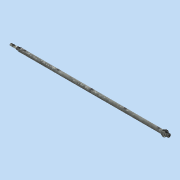
# Autodesk Inventor part: Spindel
Saved by Autodesk Inventor 2021 (Build 250183000, 183)
## iProperties
Created: 2024-03-13
Part Number: Spindel
Material: Generic
Document SubType Name: Modeling
Designer: Nokia
Density: 1 g/cm^3
Appearance: Formwork Holes
Author: Nokia
Autodesk Inventor part; units mm, degrees
ref_plane "YZ Plane" through (0, 0, 0) normal (1, 0, 0) x (0, 1, 0)
ref_plane "XZ Plane" through (0, 0, 0) normal (0, 1, 0) x (-1, 0, 0)
ref_plane "XY Plane" through (0, 0, 0) normal (0, 0, 1) x (1, 0, 0)
sketch "Sketch1" plane through (0, 0, 0) normal (0, 0, 1) x (1, 0, 0)
  line L0 (-1227.0505, 16) -> (-1227.0505, 12.5)
  arc A0 (72.9495, 16) -> (73.9495, 16) centre (73.4495, 16) ccw
  line L1 (73.9495, 16) -> (73.9495, 20)
  line L2 (73.9495, 20) -> (85.9495, 20)
  arc A1 (85.9495, 20) -> (86.9495, 20) centre (86.4495, 20) ccw
  line L3 (86.9495, 20) -> (86.9495, 26)
  line L4 (86.9495, 26) -> (98.9495, 26)
  line L5 (98.9495, 26) -> (98.9495, 15)
  arc A2 (98.9495, 15) -> (99.9495, 15) centre (99.4495, 15) ccw
  line L6 (99.9495, 15) -> (113.9495, 15)
  line L7 (-1310.4505, 0) -> (129.9495, 0)
  line L8 (-1598.5305, 0) -> (418.0295, 0) projected
  arc A3 (113.9495, 15) -> (114.9495, 15) centre (114.4495, 15) ccw
  line L9 (114.9495, 15) -> (129.9495, 15)
  line L10 (129.9495, 15) -> (129.9495, 0)
  arc A4 (-1228.0505, 12.5) -> (-1227.0505, 12.5) centre (-1227.5505, 12.5) ccw
  line L11 (-1228.0505, 12.5) -> (-1238.0505, 12.5)
  arc A5 (-1239.0505, 12.5) -> (-1238.0505, 12.5) centre (-1238.5505, 12.5) ccw
  line L12 (-1239.0505, 12.5) -> (-1251.0505, 12.5)
  line L13 (-1251.0505, 12.5) -> (-1251.0505, 10)
  line L14 (-1251.0505, 10) -> (-1310.4505, 10)
  line L15 (-1310.4505, 10) -> (-1310.4505, 0)
  arc A6 (-1219.0505, 16) -> (-1218.0505, 16) centre (-1218.5505, 16) ccw
  line L16 (72.9495, 16) -> (-1218.0505, 16)
  line L17 (-1227.0505, 16) -> (-1219.0505, 16)
  point P0 (0, 0)
  dimension "d6" = 12
  dimension "d9" = 12
  dimension "d29" = 0.5
  dimension "d30" = 0.5
  dimension "d32" = 15
  dimension "d44" = 20
  dimension "d46" = 26
  dimension "d52" = 15
  dimension "d57" = 0.5
  dimension "d58" = 10
  dimension "d62" = 2.5
  dimension "d63" = 59.4
  dimension "d70" = 1300
  dimension "d104" = 10
  dimension "d105" = 12.5
  dimension "d106" = 12.5
  dimension "d111" = 1291
  dimension "d112" = 0.5
  dimension "d113" = 0.5
  dimension "d114" = 4
  dimension "d121" = 0.5
  dimension "d122" = 0.5
  dimension "d123" = 31
  constraints: 34 end point, 14 point on circle, 7 centre point, 7 horizontal, 5 perpendicular, 4 point on line, 3 vertical
  measures "d6" distance of L1.end L2.end
  measures "d9" distance of L3.end L4.end
  measures "d29" radius of A2
  measures "d30" radius of A1
  measures "d32" distance of L9.start L9.end
  measures "d44" distance between parallel lines of L7 L2
  measures "d46" distance between parallel lines of L7 L4
  measures "d52" distance between parallel lines of L8 L9
  measures "d57" radius of A4
  measures "d58" distance of L11.start L11.end
  measures "d62" distance of L12.end L13.end
  measures "d63" distance of L13.end L14.end
  measures "d70" distance of L16.start L0.start
  measures "d104" distance of L14.end L7.start
  measures "d105" distance between parallel lines of L8 L11
  measures "d106" distance from line of L8 A4.centre
  measures "d111" distance of L16.start L16.end
  measures "d112" radius of A6
  measures "d113" radius of A0
  measures "d114" distance of L1.start L1.end
  measures "d121" radius of A5
  measures "d122" radius of A3
  measures "d123" distance between parallel lines of L5 L10
revolve "Revolution2" add sketch "Sketch1" angle 360 about axis through (-10, 0, 0) along (1, 0, 0)
chamfer "Chamfer1" distance 2 angle 45 2 edges at (98.9495, -26, 0) (86.9495, -26, 0)
thread "Thread2" size "M36x4" class "6g" standard "ANSI Metric M Profile" full length
chamfer "Chamfer2" distance 2 angle 45 1 edges at (129.9495, -15, 0)
sketch "Sketch4" plane through (129.9495, 0, 0) normal (1, 0, 0) x (0, 0, -1)
  circle A0 centre (0, 0) radius 15 projected
  line L0 (-2.5, 15) -> (2.5, 15)
  line L1 (2.5, 15) -> (2.5, 11)
  line L2 (2.5, 11) -> (-2.5, 11)
  line L3 (-2.5, 11) -> (-2.5, 15)
  point P0 (2.5, 14.7902)
  point P1 (-2.5, 14.7902)
  dimension "d47" = 4
  dimension "d49" = 5
  constraints: 8 end point, 2 horizontal, 2 perpendicular, 1 tangent
  measures "d47" distance of L0.end L1.end
  measures "d49" distance of L1.end L2.end
extrude "Extrusion3" cut sketch "Sketch4" against normal blind 16 contours L1 L2 L3 A0 picked at (0, 12.3333)
thread "Thread4" size "M30x3.5" class "6g" standard "ANSI Metric M Profile" full length
thread "Thread5" size "M25x2" class "6g" standard "ANSI Metric M Profile" full length
sketch "Sketch5" plane through (-1251.0505, 0, 0) normal (-1, 0, 0) x (0, 0, 1)
  circle A0 centre (0, 0) radius 12.5 projected
  line L0 (-2.5, 12.5) -> (2.5, 12.5)
  line L1 (2.5, 12.5) -> (2.5, 9.5)
  line L2 (2.5, 9.5) -> (-2.5, 9.5)
  line L3 (-2.5, 9.5) -> (-2.5, 12.5)
  line L4 (-2.5, 12.7574) -> (-2.5, 11) projected
  point P0 (2.5, 12.2474)
  point P1 (-2.5, 12.2474)
  dimension "d66" = 3
  dimension "d67" = 5
  constraints: 8 end point, 1 horizontal, 1 perpendicular, 1 point on line, 1 tangent
  measures "d66" distance of L0.end L1.end
  measures "d67" distance of L1.end L2.end
extrude "Extrusion4" cut sketch "Sketch5" against normal blind 13 contours L1 L2 L3 A0 picked at (0, 10.5)
chamfer "Chamfer4" distance 1 angle 45 1 edges at (73.9495, -20, 0)
chamfer "Chamfer5" distance 2 angle 45 1 edges at (-1310.4505, -10, 0)
ref_plane "Work Plane2" through (-1251.0505, 10, 0) normal (0, 1, 0) x (-1, 0, 0)
sketch "Sketch8" plane through (-1251.0505, 10, 0) normal (0, 1, 0) x (-1, 0, 0)
  line L0 (0, 10) -> (0, -10) projected
  line L1 (0, 0) -> (46.375, 0)
  line L2 (46.375, 0) -> (50.375, 0)
  arc A0 (50.375, -2) -> (50.375, 2) centre (50.375, 0) ccw
  line L3 (50.375, -2) -> (46.375, -2)
  line L4 (50.375, 2) -> (46.375, 2)
  arc A1 (42.375, 2) -> (42.375, -2) centre (42.375, 0) ccw
  line L5 (42.375, -2) -> (46.375, -2)
  line L6 (42.375, 2) -> (46.375, 2)
  point P0 (-1251.0505, 0)
  point P1 (0, 2.5)
  point P2 (0, -2.5)
  dimension "d96" = 4
  dimension "d97" = 4
  constraints: 12 end point, 6 point on circle, 2 centre point, 2 horizontal, 1 coincident, 1 midpoint, 1 other
  measures "d96" distance of L1.end L2.end
  measures "d97" diameter of A0
extrude "Extrusion5" cut sketch "Sketch8" against normal blind 3
fillet "Fillet1" radius 0.25 4 edges at (-1297.4255, 7, -2) (-1291.4255, 7, 0) (-1297.4255, 7, 2) (-1303.4255, 7, 0)
chamfer "Chamfer6" distance 0.25 angle 45 6 edges at (-1297.4255, 9.798, -2) (-1292.1196, 9.8846, -1.5148) (-1292.1204, 9.8845, 1.5155) (-1297.4255, 9.798, 2) (-1302.7314, 9.8846, 1.5148) (-1302.7306, 9.8845, -1.5155)
chamfer "Chamfer7" distance 2 angle 45 1 edges at (-1251.0505, -12.5, 0)
chamfer "Chamfer8" distance 1 angle 45 1 edges at (-1227.0505, -16, 0)
body "Solid2"
